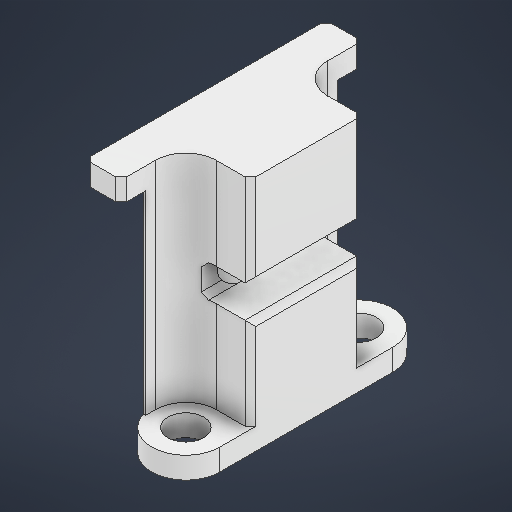
# Autodesk Inventor part: CNC-026-CableCarrierTrack
Saved by Autodesk Inventor 2026.2 (Build 302298000, 298)
## iProperties
Created: 2026-06-25
Part Number: CNC-026-CableCarrierTrack
Material: ABS Plastic
Document SubType Name: Modeling
Designer: Kenji
Density: 1.06 g/cm^3
Appearance: Smooth - White
Author: Kenji
Autodesk Inventor part; units mm, degrees
ref_plane "YZ Plane" through (0, 0, 0) normal (1, 0, 0) x (0, 1, 0)
ref_plane "XZ Plane" through (0, 0, 0) normal (0, 1, 0) x (-1, 0, 0)
ref_plane "XY Plane" through (0, 0, 0) normal (0, 0, 1) x (1, 0, 0)
sketch "Sketch1" plane through (0, 0, 0) normal (0, 1, 0) x (-1, 0, 0)
  circle A0 centre (0, 0) radius 2.63
  circle A1 centre (0, 0) radius 5 construction
  circle A2 centre (0, -25.4) radius 2.63
  circle A3 centre (0, -25.4) radius 5 construction
  line L0 (5, -25.4) -> (5, 0)
  line L1 (-5, 0) -> (-5, -25.4)
  arc A4 (-5, -25.4) -> (5, -25.4) centre (0, -25.4) ccw
  arc A5 (5, 0) -> (-5, 0) centre (0, 0) ccw
  point P0 (2.63, 0)
  dimension "d0" = 5.26
  dimension "d1" = 2.37
  dimension "d2" = 25.4
  constraints: 8 point on circle, 6 tangent, 5 centre point, 4 end point, 3 coincident, 3 horizontal alignment, 1 concentric, 1 equal radius, 1 vertical, 1 vertical alignment, 3 other
  measures "d1" distance of point (2.63, 0) L0.end
  measures "d2" distance of A2.centre point (0, 0)
extrude "Extrusion1" add sketch "Sketch1" along normal blind 31.75
sketch "Sketch2" plane through (0, 31.75, 0) normal (0, 1, 0) x (1, 0, 0)
  arc A0 (-5, 0) -> (5, 0) centre (0, 0) ccw projected
  line L0 (5, 0) -> (5, 25.4) projected
  arc A1 (5, 25.4) -> (-5, 25.4) centre (0, 25.4) ccw projected
  line L1 (-5, 25.4) -> (-5, 0) projected
  circle A2 centre (0, 25.4) radius 2.63 projected
  circle A3 centre (0, 0) radius 2.63 projected
  line L2 (0, -5) -> (-6.5875, -5)
  line L3 (-9.7625, -1.825) -> (-9.7625, 27.225)
  line L4 (-6.5875, 30.4) -> (0, 30.4)
  arc A4 (-9.7625, -1.825) -> (-6.5875, -5) centre (-6.5875, -1.825) ccw
  arc A5 (-6.5875, 30.4) -> (-9.7625, 27.225) centre (-6.5875, 27.225) ccw
  dimension "d5" = 4.7625
  dimension "d6" = 3.175
  constraints: 6 end point, 6 point on circle, 6 tangent, 2 centre point, 2 perpendicular, 1 equal radius, 1 horizontal
  measures "d5" distance between parallel lines of L1 L3
  measures "d6" radius of A4
extrude "Extrusion2" add sketch "Sketch2" along normal blind 3.175
sketch "Sketch3" plane through (0, 34.925, 0) normal (0, 1, 0) x (1, 0, 0)
  circle A0 centre (0, 0) radius 4.5
  circle A1 centre (0, 25.4) radius 2.63 projected
  circle A2 centre (0, 25.4) radius 4.5
  dimension "d9" = 9
  constraints: 2 centre point, 2 coincident, 1 equal radius
  measures "d9" diameter of A0
extrude "Extrusion3" cut sketch "Sketch3" against normal blind 31.75
sketch "Sketch4" plane through (0, 34.925, 0) normal (0, 1, 0) x (1, 0, 0)
  circle A0 centre (0, 25.4) radius 4.5 projected
  circle A1 centre (0, 0) radius 4.5 projected
  arc A2 (-6.5875, 30.4) -> (-9.7625, 27.225) centre (-6.5875, 27.225) ccw projected
  line L0 (-9.7625, 27.225) -> (-9.7625, -1.825) projected
  arc A3 (-9.7625, -1.825) -> (-6.5875, -5) centre (-6.5875, -1.825) ccw projected
  line L1 (-6.5875, -5) -> (0, -5) projected
  arc A4 (0, -5) -> (5, 0) centre (0, 0) ccw projected
  line L2 (5, 0) -> (5, 25.4) projected
  arc A5 (5, 25.4) -> (0, 30.4) centre (0, 25.4) ccw projected
  line L3 (0, 30.4) -> (-6.5875, 30.4) projected
  line L4 (0, 20.9) -> (5, 20.9)
  circle A6 centre (0, 25.4) radius 4.5 projected
  line L5 (-4.5, 25.4) -> (-4.5, 30.4)
  line L6 (0, 4.5) -> (5, 4.5)
  line L7 (-4.5, 0) -> (-4.5, -5)
  constraints: 8 end point, 6 point on line, 3 perpendicular, 3 point on circle, 3 tangent, 1 vertical, 2 other
extrude "Extrusion4" cut sketch "Sketch4" against normal blind 31.75 contours A0 L5 L3 A5 L2 L4 | L2 A4 L1 L7 A1 L6
sketch "Sketch5" plane through (-5, 0, -25.4) normal (-1, 0, 0) x (0, 0, 1)
  circle A0 centre (8.89, 19.05) radius 2.38125
  circle A1 centre (16.51, 19.05) radius 2.38125
  line L0 (-1.825, 34.925) -> (27.225, 34.925)
  line L1 (27.579449, 3.175) -> (27.579449, 31.75)
  line L2 (-2.179449, 31.75) -> (-2.179449, 3.175)
  point P0 (25.4, 0)
  dimension "d14" = 4.7625
  dimension "d15" = 7.62
  dimension "d16" = 15.875
  dimension "d17" = 29.7589
  dimension "d18" = 11.06945
  constraints: 2 centre point, 1 equal radius, 1 horizontal alignment
  measures "d14" diameter of A0
  measures "d15" distance of A0.centre A1.centre
  measures "d16" distance from line of L0 A0.centre
  measures "d17" distance between parallel lines of L1 L2
  measures "d18" distance from line of A0.centre L2
extrude "Extrusion5" cut sketch "Sketch5" against normal through all
sketch "Sketch6" plane through (5, 0, 0) normal (1, 0, 0) x (0, 0, -1)
  circle A0 centre (8.89, 19.05) radius 2.38125
  circle A1 centre (16.51, 19.05) radius 2.38125
  line L0 (20.9, 3.175) -> (20.9, 34.925)
  line L1 (4.5, 34.925) -> (20.9, 34.925)
  line L2 (4.5, 34.925) -> (4.5, 3.175)
  line L3 (0, 0) -> (0, 3.175)
  line L4 (0, 0) -> (25.4, 0)
  line L5 (25.4, 0) -> (25.4, 3.175)
  circle A2 centre (16.51, 19.05) radius 2.38125
  line L6 (16.51, 21.43125) -> (8.89, 21.43125)
  line L7 (16.51, 16.66875) -> (8.89, 16.66875)
  line L8 (4.5, 3.175) -> (0, 3.175)
  line L9 (25.4, 3.175) -> (20.9, 3.175)
  constraints: 5 tangent, 4 end point, 4 point on circle
extrude "Extrusion6" cut sketch "Sketch6" against normal blind 6.8326 contours A0 L6 A1 L7
sketch "Sketch7" plane through (0, 34.925, 0) normal (0, 1, 0) x (1, 0, 0)
  line L0 (5, 20.9) -> (0, 20.9) projected
  arc A0 (-4.5, 25.4) -> (0, 20.9) centre (0, 25.4) ccw projected
  line L1 (-4.5, 25.4) -> (-4.5, 30.4) projected
  line L2 (-4.5, 30.4) -> (-6.5875, 30.4) projected
  arc A1 (-6.5875, 30.4) -> (-9.7625, 27.225) centre (-6.5875, 27.225) ccw projected
  line L3 (-9.7625, 27.225) -> (-9.7625, -1.825) projected
  arc A2 (-9.7625, -1.825) -> (-6.5875, -5) centre (-6.5875, -1.825) ccw projected
  line L4 (-6.5875, -5) -> (-4.5, -5) projected
  line L5 (-4.5, -5) -> (-4.5, 0) projected
  arc A3 (0, 4.5) -> (-4.5, 0) centre (0, 0) ccw projected
  line L6 (0, 4.5) -> (5, 4.5) projected
  line L7 (5, 4.5) -> (5, 20.9) projected
  line L8 (-6.5875, -5) -> (-9.7625, -5)
  arc A4 (-9.7625, -1.825) -> (-6.5875, -5) centre (-6.5875, -1.825) ccw projected
  line L9 (-9.7625, 27.225) -> (-9.7625, -1.825) projected
  line L10 (-9.7625, -5) -> (-9.7625, -1.825)
  line L11 (-9.7625, 27.225) -> (-9.7625, 30.4)
  arc A5 (-6.5875, 30.4) -> (-9.7625, 27.225) centre (-6.5875, 27.225) ccw projected
  line L12 (-9.7625, 30.4) -> (-6.5875, 30.4)
  constraints: 8 end point, 4 tangent, 1 collinear, 1 horizontal, 1 perpendicular, 1 vertical
extrude "Extrusion7" add sketch "Sketch7" against normal up to surface (3.175 mm away) contours A1 L11 L12 | L8 L10 A2
chamfer "Chamfer1" distance 0.79375 angle 45 6 edges at (-9.7625, 33.3375, 5) (-4.5, 33.3375, 5) (-4.5, 33.3375, -30.4) (-9.7625, 33.3375, -30.4) (-4.5, 17.4625, -27.5794) (-4.5, 17.4625, 2.1794)
chamfer "Chamfer2" distance 0.79375 angle 45 2 edges at (5, 19.05, -4.5) (5, 19.05, -20.9)
sketch "Sketch8" plane through (5, 0, 0) normal (1, 0, 0) x (0, 0, -1)
  line L0 (25.4, 3.175) -> (20.10625, 3.175)
  line L1 (20.10625, 34.925) -> (20.10625, 3.175)
  line L2 (5.29375, 34.925) -> (20.10625, 34.925)
  line L3 (5.29375, 3.175) -> (5.29375, 34.925)
  line L4 (5.29375, 3.175) -> (0, 3.175)
  line L5 (0, 0) -> (0, 3.175)
  line L6 (0, 0) -> (25.4, 0)
  line L7 (25.4, 0) -> (25.4, 3.175)
  line L8 (8.89, 21.43125) -> (16.51, 21.43125)
  arc A0 (16.51, 16.66875) -> (16.51, 21.43125) centre (16.51, 19.05) ccw
  line L9 (16.51, 16.66875) -> (8.89, 16.66875)
  arc A1 (8.89, 21.43125) -> (8.89, 16.66875) centre (8.89, 19.05) ccw
  line L10 (4.5, 34.925) -> (4.5, 3.175)
  line L11 (20.9, 3.175) -> (20.9, 34.925)
  line L12 (8.89, 16.66875) -> (-1.385699, 16.66875)
  line L13 (-1.385699, 3.175) -> (-1.385699, 31.75)
  line L14 (8.89, 21.43125) -> (-1.385699, 21.43125)
  line L15 (16.51, 21.43125) -> (26.785699, 21.43125)
  line L16 (26.785699, 31.75) -> (26.785699, 3.175)
  line L17 (16.51, 16.66875) -> (26.785699, 16.66875)
  constraints: 8 end point, 4 horizontal, 3 point on line
extrude "Extrusion8" cut sketch "Sketch8" against normal up to surface (6.8326 mm away) contours L17 L1 L15 L11 | L11 L15 L16 L17 | L17 A0 L15 L1 | L12 L3 L14 A1 | L12 L13 L14 L10 | L10 L14 L3 L12
chamfer "Chamfer3" distance 0.79375 angle 45 8 edges at (5, 16.6687, -12.7) (5, 21.4312, -12.7) (-1.8326, 16.6687, -6.5) (-1.8326, 16.6687, -12.7) (-1.8326, 16.6687, -18.9) (-1.8326, 21.4312, -6.5) (-1.8326, 21.4312, -12.7) (-1.8326, 21.4312, -18.9)
equation "\"d18\" = 0.5 * d17 - 0.5 * d15"
body "Solid1"
